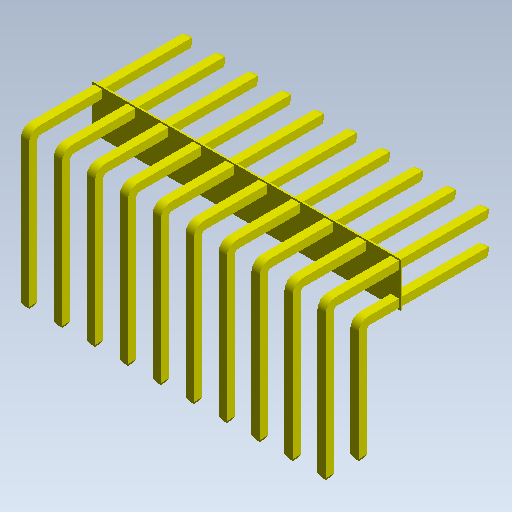
# Autodesk Inventor part: T-1S6-09-TSW-1-09-10-RA-D
Saved by Autodesk Inventor 2021 (Build 250183000, 183)
## iProperties
Part Number: T-1S6-09-TSW-1-09-10-RA-D
Material: Generic
Catalog Web Link: www.cadenas.de
Description: TSW Series Pin-TSW Series - (2,54 mm) .100" Through-Hole .025" Square Post Header
Vendor: SAMTEC
Document SubType Name: Modeling
Designer: partserver
Manufacturer: SAMTEC
Mass: 0.179842 g
Surface Area: 12.3232 cm^2
Volume: 0.179842 cm^3
Density: 1 g/cm^3
Appearance: PSOLRGB-255-255-0
Category: PARTsolutions
Company: SAMTEC
PSOL_IDENT_0: {$CADENAS_DATA\23d-libs\samtec\modelling\tsw\parts\tsw_pin.prj},230 {VTYP=3D},{NB=T-1S6-09-TSW-1-09-
PSOL_IDENT_1: 10-RA-D},{LINA=T-1S6-09-TSW-1-09-10-RA-D},{NN=TSW Series Pin},{DATE=29.08.2019 09:17:37},{GEOMDATE=1
PSOL_IDENT_2: 0.06.2019 10:17:41},{VERSION=},{LINEID=50},{WBVAR=TSS,POS,TOPT,ROW,POLOPT,LLOPT},{WBNUMERIC=POS}  {N
PSOL_IDENT_3: B=T-1S6-09-TSW-1-09-10-RA-D},{LINA=T-1S6-09-TSW-1-09-10-RA-D},{KT=DUMMY},{PN=T-1S6-09},{TSS=-1},{POS=
PSOL_IDENT_4: 10},{TOPT=-RA},{TOPTALG= '','Straight Body' , '-RA','-RA - Right Angle' , '-NA','-NA - Right Angle w
PSOL_IDENT_5: ith Straight Body' , '-LA','-LA - Right Angle with Locking Lead' },{ROW=-D},{ROWALG= '-S','-S - Sing
PSOL_IDENT_6: le','-D','-D - Double','-T','-T - Triple','-Q','-Q - Triple (Fill Outer Rows only)' },{POLOPT=},{POL
PSOL_IDENT_7: OPTALG= '','Not Selected','001','001','002','002','003','003','004','004','005','005','006','006','0
PSOL_IDENT_8: 07','007','008','008','009','009','010','010','011','011','012','012','013','013','014','014','015','
PSOL_IDENT_9: 015','016','016','017','017','018','018','019','019','020','020' },{POLOPTMAX=240},{POLOPTMAX2='001'
PSOL_IDENT_10: ,'001','002','002','003','003','004','004','005','005','006','006','007','007','008','008','009','00
PSOL_IDENT_11: 9','010','010','011','011','012','012','013','013','014','014','015','015','016','016','017','017','
PSOL_IDENT_12: 018','018','019','019','020','020'},{POLARIZE='001','001','002','002','003','003','004','004','005','
PSOL_IDENT_13: 005','006','006','007','007','008','008','009','009','010','010','011','011','012','012','013','013'
PSOL_IDENT_14: ,'014','014','015','015','016','016','017','017','018','018','019','019','020','020','021','021','02
PSOL_IDENT_15: 2','022','023','023','024','024','025','025','026','026','027','027','028','028','029','029','030','
PSOL_IDENT_16: 030','031','031','032','032','033','033','034','034','035','035','036','036','037','037','038','038'
PSOL_IDENT_17: ,'039','039','040','040','041','041','042','042','043','043','044','044','045','045','046','046','04
PSOL_IDENT_18: 7','047','048','048','049','049','050','050','051','051','052','052','053','053','054','054','055','
PSOL_IDENT_19: 055','056','056','057','057','058','058','059','059','060','060','061','061','062','062','063','063'
PSOL_IDENT_20: ,'064','064','065','065','066','066','067','067','068','068','069','069','070','070','071','071','07
PSOL_IDENT_21: 2','072','073','073','074','074','075','075','076','076','077','077','078','078','079','079','080','
PSOL_IDENT_22: 080','081','081','082','082','083','083','084','084','085','085','086','086','087','087','088','088'
PSOL_IDENT_23: ,'089','089','090','090','091','091','092','092','093','093','094','094','095','095','096','096','09
PSOL_IDENT_24: 7','097','098','098','099','099','100','100','101','101','102','102','103','103','104','104','105','
PSOL_IDENT_25: 105','106','106','107','107','108','108','109','109','110','110','111','111','112','112','113','113'
PSOL_IDENT_26: ,'114','114','115','115','116','116','117','117','118','118','119','119','120','120','121','121','12
PSOL_IDENT_27: 2','122','123','123','124','124','125','125','126','126','127','127','128','128','129','129','130','
PSOL_IDENT_28: 130','131','131','132','132','133','133','134','134','135','135','136','136','137','137','138','138'
PSOL_IDENT_29: ,'139','139','140','140','141','141','142','142','143','143','144','144','145','145','146','146','14
PSOL_IDENT_30: 7','147','148','148','149','149','150','150'},{POLOPTATOF=0},{POLOPTPN=},{LLOPT=},{LLOPTALG= '','Not
PSOL_IDENT_31: Selected','-LL','-LL - Locking Lead' },{POLOE=0},{LS=-09},{AS=0.400},{BS=0.730},{CS=0.230},{ARA=0.2
PSOL_IDENT_32: 90},{ARE=0.190},{ANA=0.309},{ANE=0.209},{BRANA=0.060},{BRENE=0.160},{CRANA=0.230},{CRENE=0.230},{BW=
PSOL_IDENT_33: 0.20000},{PM=1.00000},{PP=-0.06250},{A=1.00000},{POLPX=-0.4375},{POLPY=0.0000},{POL3DB=0},{POSOE=2},
PSOL_IDENT_34: {LLP=0.050},{D=0.060},{ST= '','Straight Body' },{RA= '-RA','-RA - Right Angle' },{RE=},{NA= '-NA','-
PSOL_IDENT_35: NA - Right Angle with Straight Body' },{NE=},{LA= '-LA','-LA - Right Angle with Locking Lead' },{AP=
PSOL_IDENT_36: 0.290},{BP=0.06},{CP=0.230},{BW2=0.160}
NB: T-1S6-09-TSW-1-09-10-RA-D
NN: TSW Series Pin
NT: TSW Series - (2,54 mm) .100" Through-Hole .025" Square Post Header
NBSYN: $PN.-TSW$TSS.$LS.-$POS.$TOPT.$ROW.$POLOPTPN.$LLOPT.
LINA: T-1S6-09-TSW-1-09-10-RA-D
CATALOG: Samtec
PN: T-1S6-09
TSS: -1 - .100 [2.54] Fill every position
POS: 10
TOPT: -RA - Right Angle
ROW: -D - Double
POLOPT: Not Selected
LLOPT: Not Selected
LS: -09
AS: 0.4
BS: 0.73
CS: 0.23
ARA: 0.29
ARE: 0.19
ANA: 0.309
ANE: 0.209
BRANA: 0.06
BRENE: 0.16
CRANA: 0.23
CRENE: 0.23
SUPPLIER: SAMTEC
ARTICLENO: T-1S6-09-TSW-1-09-10-RA-D
BOMINFO: T-1S6-09-TSW-1-09-10-RA-D
CREATOR: CADENAS GmbH
Title: T-1S6-09-TSW-1-09-10-RA-D
Author: Cadenas PARTsolutions
Comments: TSW Series - (2,54 mm) .100" Through-Hole .025" Square Post Header
Autodesk Inventor part; units mm, degrees
sketch "Sketch_1" plane through (0, 0, 0) normal (1, 0, 0) x (0, 1, 0)
  line L0 (0.1415, 10.414) -> (-0.1415, 10.414)
  line L1 (-0.1415, 10.414) -> (-0.3175, 10.1092)
  line L2 (-0.3175, 10.1092) -> (-0.3175, 1.7145)
  arc A0 (-0.3175, 1.7145) -> (0.4445, 0.9525) centre (0.4445, 1.7145) ccw
  line L3 (0.4445, 0.9525) -> (9.6012, 0.9525)
  line L4 (9.6012, 0.9525) -> (9.906, 1.1285)
  line L5 (9.906, 1.1285) -> (9.906, 1.4115)
  line L6 (9.906, 1.4115) -> (9.6012, 1.5875)
  line L7 (9.6012, 1.5875) -> (0.5715, 1.5875)
  arc A1 (0.3175, 1.8415) -> (0.5715, 1.5875) centre (0.5715, 1.8415) ccw
  line L8 (0.3175, 1.8415) -> (0.3175, 10.1092)
  line L9 (0.3175, 10.1092) -> (0.1415, 10.414)
  constraints: 20 end point, 4 point on circle, 2 centre point
extrude "Extrusion1" add sketch "Sketch_1" along normal mid plane 23.495
sketch "Sketch_36" plane through (0, 0, 0) normal (1, 0, 0) x (0, 1, 0)
  line L0 (-2.3985, 10.414) -> (-2.6815, 10.414)
  line L1 (-2.6815, 10.414) -> (-2.8575, 10.1092)
  line L2 (-2.8575, 10.1092) -> (-2.8575, -0.8255)
  arc A0 (-2.8575, -0.8255) -> (-2.0955, -1.5875) centre (-2.0955, -0.8255) ccw
  line L3 (-2.0955, -1.5875) -> (9.6012, -1.5875)
  line L4 (9.6012, -1.5875) -> (9.906, -1.4115)
  line L5 (9.906, -1.4115) -> (9.906, -1.1285)
  line L6 (9.906, -1.1285) -> (9.6012, -0.9525)
  line L7 (9.6012, -0.9525) -> (-1.9685, -0.9525)
  arc A1 (-2.2225, -0.6985) -> (-1.9685, -0.9525) centre (-1.9685, -0.6985) ccw
  line L8 (-2.2225, -0.6985) -> (-2.2225, 10.1092)
  line L9 (-2.2225, 10.1092) -> (-2.3985, 10.414)
  constraints: 20 end point, 4 point on circle, 2 centre point
sketch "Sketch_26" plane through (0, 0, 0) normal (1, 0, 0) x (0, 1, 0)
  line L0 (2.921, 1.7145) -> (2.794, 1.7145)
  line L1 (2.794, 1.7145) -> (2.794, -1.7145)
  line L2 (2.794, -1.7145) -> (2.921, -1.7145)
  line L3 (2.921, -1.7145) -> (2.921, 1.7145)
  constraints: 8 end point
extrude "Extrusion2" add sketch "Sketch_26" along normal mid plane 23.749
extrude "Extrusion3" add sketch "Sketch_36" along normal mid plane 23.495
sketch "Sketch_9" plane through (0, 0, 0) normal (0, 0, 1) x (1, 0, 0)
  line L0 (-11.1125, 17.653) -> (-11.1125, 2.921)
  line L1 (-11.1125, 2.921) -> (-9.2075, 2.921)
  line L2 (-9.2075, 2.921) -> (-9.2075, 10.2235)
  line L3 (-9.2075, 10.2235) -> (-8.5725, 10.2235)
  line L4 (-8.5725, 10.2235) -> (-8.5725, 2.921)
  line L5 (-8.5725, 2.921) -> (-6.6675, 2.921)
  line L6 (-6.6675, 2.921) -> (-6.6675, 10.2235)
  line L7 (-6.6675, 10.2235) -> (-6.0325, 10.2235)
  line L8 (-6.0325, 10.2235) -> (-6.0325, 2.921)
  line L9 (-6.0325, 2.921) -> (-4.1275, 2.921)
  line L10 (-4.1275, 2.921) -> (-4.1275, 10.2235)
  line L11 (-4.1275, 10.2235) -> (-3.4925, 10.2235)
  line L12 (-3.4925, 10.2235) -> (-3.4925, 2.921)
  line L13 (-3.4925, 2.921) -> (-1.5875, 2.921)
  line L14 (-1.5875, 2.921) -> (-1.5875, 10.2235)
  line L15 (-1.5875, 10.2235) -> (-0.9525, 10.2235)
  line L16 (-0.9525, 10.2235) -> (-0.9525, 2.921)
  line L17 (-0.9525, 2.921) -> (0.9525, 2.921)
  line L18 (0.9525, 2.921) -> (0.9525, 10.2235)
  line L19 (0.9525, 10.2235) -> (1.5875, 10.2235)
  line L20 (1.5875, 10.2235) -> (1.5875, 2.921)
  line L21 (1.5875, 2.921) -> (3.4925, 2.921)
  line L22 (3.4925, 2.921) -> (3.4925, 10.2235)
  line L23 (3.4925, 10.2235) -> (4.1275, 10.2235)
  line L24 (4.1275, 10.2235) -> (4.1275, 2.921)
  line L25 (4.1275, 2.921) -> (6.0325, 2.921)
  line L26 (6.0325, 2.921) -> (6.0325, 10.2235)
  line L27 (6.0325, 10.2235) -> (6.6675, 10.2235)
  line L28 (6.6675, 10.2235) -> (6.6675, 2.921)
  line L29 (6.6675, 2.921) -> (8.5725, 2.921)
  line L30 (8.5725, 2.921) -> (8.5725, 10.2235)
  line L31 (8.5725, 10.2235) -> (9.2075, 10.2235)
  line L32 (9.2075, 10.2235) -> (9.2075, 2.921)
  line L33 (9.2075, 2.921) -> (11.1125, 2.921)
  line L34 (11.1125, 2.921) -> (11.1125, 17.653)
  line L35 (11.1125, 17.653) -> (-11.1125, 17.653)
  constraints: 72 end point
extrude "Extrusion4" cut sketch "Sketch_9" along normal mid plane 10.16
sketch "Sketch_12" plane through (0, 0, 0) normal (0, 0, 1) x (1, 0, 0)
  line L0 (-11.1125, -48.006) -> (11.1125, -48.006)
  line L1 (11.1125, -48.006) -> (11.1125, 2.794)
  line L2 (11.1125, 2.794) -> (9.2075, 2.794)
  line L3 (9.2075, 2.794) -> (9.2075, -5.588)
  line L4 (9.2075, -5.588) -> (8.5725, -5.588)
  line L5 (8.5725, -5.588) -> (8.5725, 2.794)
  line L6 (8.5725, 2.794) -> (6.6675, 2.794)
  line L7 (6.6675, 2.794) -> (6.6675, -5.588)
  line L8 (6.6675, -5.588) -> (6.0325, -5.588)
  line L9 (6.0325, -5.588) -> (6.0325, 2.794)
  line L10 (6.0325, 2.794) -> (4.1275, 2.794)
  line L11 (4.1275, 2.794) -> (4.1275, -5.588)
  line L12 (4.1275, -5.588) -> (3.4925, -5.588)
  line L13 (3.4925, -5.588) -> (3.4925, 2.794)
  line L14 (3.4925, 2.794) -> (1.5875, 2.794)
  line L15 (1.5875, 2.794) -> (1.5875, -5.588)
  line L16 (1.5875, -5.588) -> (0.9525, -5.588)
  line L17 (0.9525, -5.588) -> (0.9525, 2.794)
  line L18 (0.9525, 2.794) -> (-0.9525, 2.794)
  line L19 (-0.9525, 2.794) -> (-0.9525, -5.588)
  line L20 (-0.9525, -5.588) -> (-1.5875, -5.588)
  line L21 (-1.5875, -5.588) -> (-1.5875, 2.794)
  line L22 (-1.5875, 2.794) -> (-3.4925, 2.794)
  line L23 (-3.4925, 2.794) -> (-3.4925, -5.588)
  line L24 (-3.4925, -5.588) -> (-4.1275, -5.588)
  line L25 (-4.1275, -5.588) -> (-4.1275, 2.794)
  line L26 (-4.1275, 2.794) -> (-6.0325, 2.794)
  line L27 (-6.0325, 2.794) -> (-6.0325, -5.588)
  line L28 (-6.0325, -5.588) -> (-6.6675, -5.588)
  line L29 (-6.6675, -5.588) -> (-6.6675, 2.794)
  line L30 (-6.6675, 2.794) -> (-8.5725, 2.794)
  line L31 (-8.5725, 2.794) -> (-8.5725, -5.588)
  line L32 (-8.5725, -5.588) -> (-9.2075, -5.588)
  line L33 (-9.2075, -5.588) -> (-9.2075, 2.794)
  line L34 (-9.2075, 2.794) -> (-11.1125, 2.794)
  line L35 (-11.1125, 2.794) -> (-11.1125, -48.006)
  constraints: 72 end point
extrude "Extrusion5" cut sketch "Sketch_12" along normal mid plane 508
sketch "Sketch_33" plane through (0, 0, 0) normal (0, 0, 1) x (1, 0, 0)
  line L0 (-11.7475, 9.6012) -> (-11.5715, 9.906)
  line L1 (-11.5715, 9.906) -> (-11.2885, 9.906)
  line L2 (-11.2885, 9.906) -> (-11.1125, 9.6012)
  line L3 (-11.1125, 9.6012) -> (-9.2075, 9.6012)
  line L4 (-9.2075, 9.6012) -> (-9.0315, 9.906)
  line L5 (-9.0315, 9.906) -> (-8.7485, 9.906)
  line L6 (-8.7485, 9.906) -> (-8.5725, 9.6012)
  line L7 (-8.5725, 9.6012) -> (-6.6675, 9.6012)
  line L8 (-6.6675, 9.6012) -> (-6.4915, 9.906)
  line L9 (-6.4915, 9.906) -> (-6.2085, 9.906)
  line L10 (-6.2085, 9.906) -> (-6.0325, 9.6012)
  line L11 (-6.0325, 9.6012) -> (-4.1275, 9.6012)
  line L12 (-4.1275, 9.6012) -> (-3.9515, 9.906)
  line L13 (-3.9515, 9.906) -> (-3.6685, 9.906)
  line L14 (-3.6685, 9.906) -> (-3.4925, 9.6012)
  line L15 (-3.4925, 9.6012) -> (-1.5875, 9.6012)
  line L16 (-1.5875, 9.6012) -> (-1.4115, 9.906)
  line L17 (-1.4115, 9.906) -> (-1.1285, 9.906)
  line L18 (-1.1285, 9.906) -> (-0.9525, 9.6012)
  line L19 (-0.9525, 9.6012) -> (0.9525, 9.6012)
  line L20 (0.9525, 9.6012) -> (1.1285, 9.906)
  line L21 (1.1285, 9.906) -> (1.4115, 9.906)
  line L22 (1.4115, 9.906) -> (1.5875, 9.6012)
  line L23 (1.5875, 9.6012) -> (3.4925, 9.6012)
  line L24 (3.4925, 9.6012) -> (3.6685, 9.906)
  line L25 (3.6685, 9.906) -> (3.9515, 9.906)
  line L26 (3.9515, 9.906) -> (4.1275, 9.6012)
  line L27 (4.1275, 9.6012) -> (6.0325, 9.6012)
  line L28 (6.0325, 9.6012) -> (6.2085, 9.906)
  line L29 (6.2085, 9.906) -> (6.4915, 9.906)
  line L30 (6.4915, 9.906) -> (6.6675, 9.6012)
  line L31 (6.6675, 9.6012) -> (8.5725, 9.6012)
  line L32 (8.5725, 9.6012) -> (8.7485, 9.906)
  line L33 (8.7485, 9.906) -> (9.0315, 9.906)
  line L34 (9.0315, 9.906) -> (9.2075, 9.6012)
  line L35 (9.2075, 9.6012) -> (11.1125, 9.6012)
  line L36 (11.1125, 9.6012) -> (11.2885, 9.906)
  line L37 (11.2885, 9.906) -> (11.5715, 9.906)
  line L38 (11.5715, 9.906) -> (11.7475, 9.6012)
  line L39 (11.7475, 9.6012) -> (11.7475, 12.1412)
  line L40 (11.7475, 12.1412) -> (-11.7475, 12.1412)
  line L41 (-11.7475, 12.1412) -> (-11.7475, 9.6012)
  constraints: 84 end point
extrude "Extrusion6" cut sketch "Sketch_33" along normal mid plane 10.16
sketch "Sketch_38" plane through (0, 0, 0) normal (0, 1, 0) x (-1, 0, 0)
  line L0 (11.7475, 12.6619) -> (-11.7475, 12.6619)
  line L1 (-11.7475, 12.6619) -> (-11.7475, 10.1219)
  line L2 (-11.7475, 10.1219) -> (-11.5715, 10.4267)
  line L3 (-11.5715, 10.4267) -> (-11.2885, 10.4267)
  line L4 (-11.2885, 10.4267) -> (-11.1125, 10.1219)
  line L5 (-11.1125, 10.1219) -> (-9.2075, 10.1219)
  line L6 (-9.2075, 10.1219) -> (-9.0315, 10.4267)
  line L7 (-9.0315, 10.4267) -> (-8.7485, 10.4267)
  line L8 (-8.7485, 10.4267) -> (-8.5725, 10.1219)
  line L9 (-8.5725, 10.1219) -> (-6.6675, 10.1219)
  line L10 (-6.6675, 10.1219) -> (-6.4915, 10.4267)
  line L11 (-6.4915, 10.4267) -> (-6.2085, 10.4267)
  line L12 (-6.2085, 10.4267) -> (-6.0325, 10.1219)
  line L13 (-6.0325, 10.1219) -> (-4.1275, 10.1219)
  line L14 (-4.1275, 10.1219) -> (-3.9515, 10.4267)
  line L15 (-3.9515, 10.4267) -> (-3.6685, 10.4267)
  line L16 (-3.6685, 10.4267) -> (-3.4925, 10.1219)
  line L17 (-3.4925, 10.1219) -> (-1.5875, 10.1219)
  line L18 (-1.5875, 10.1219) -> (-1.4115, 10.4267)
  line L19 (-1.4115, 10.4267) -> (-1.1285, 10.4267)
  line L20 (-1.1285, 10.4267) -> (-0.9525, 10.1219)
  line L21 (-0.9525, 10.1219) -> (0.9525, 10.1219)
  line L22 (0.9525, 10.1219) -> (1.1285, 10.4267)
  line L23 (1.1285, 10.4267) -> (1.4115, 10.4267)
  line L24 (1.4115, 10.4267) -> (1.5875, 10.1219)
  line L25 (1.5875, 10.1219) -> (3.4925, 10.1219)
  line L26 (3.4925, 10.1219) -> (3.6685, 10.4267)
  line L27 (3.6685, 10.4267) -> (3.9515, 10.4267)
  line L28 (3.9515, 10.4267) -> (4.1275, 10.1219)
  line L29 (4.1275, 10.1219) -> (6.0325, 10.1219)
  line L30 (6.0325, 10.1219) -> (6.2085, 10.4267)
  line L31 (6.2085, 10.4267) -> (6.4915, 10.4267)
  line L32 (6.4915, 10.4267) -> (6.6675, 10.1219)
  line L33 (6.6675, 10.1219) -> (8.5725, 10.1219)
  line L34 (8.5725, 10.1219) -> (8.7485, 10.4267)
  line L35 (8.7485, 10.4267) -> (9.0315, 10.4267)
  line L36 (9.0315, 10.4267) -> (9.2075, 10.1219)
  line L37 (9.2075, 10.1219) -> (11.1125, 10.1219)
  line L38 (11.1125, 10.1219) -> (11.2885, 10.4267)
  line L39 (11.2885, 10.4267) -> (11.5715, 10.4267)
  line L40 (11.5715, 10.4267) -> (11.7475, 10.1219)
  line L41 (11.7475, 10.1219) -> (11.7475, 12.6619)
  constraints: 84 end point
extrude "Extrusion7" cut sketch "Sketch_38" along normal mid plane 20.32
ref_plane "pin_XY" through (0, 1.524, 0) normal (0, 1, 0) x (1, 0, 0)
ref_plane "pin_YZ" through (0, 1.524, 0) normal (1, 0, 0) x (0, 0, -1)
ref_plane "pin_ZX" through (0, 1.524, 0) normal (0, 0, -1) x (0, 1, 0)
body "Solid1"
